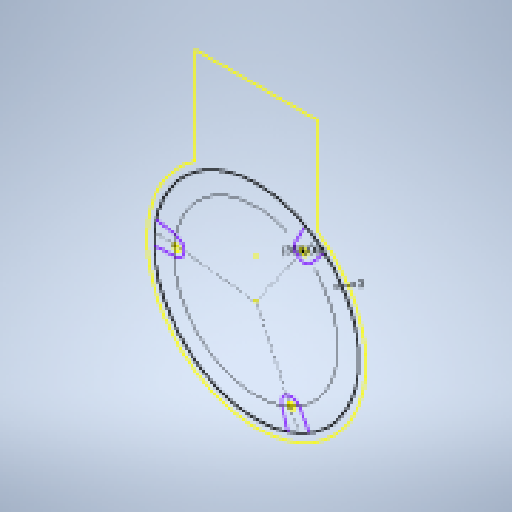
# Autodesk Inventor part: clips Anemo
Saved by Autodesk Inventor 2023 (Build 270158000, 158)
## iProperties
Created: 2023-03-28
Part Number: clips Anemo
Material: Générique
Document SubType Name: Modeling
Designer: eleves
Density: 1 g/cm^3
Appearance: Par défaut
Author: eleves
Autodesk Inventor part; units mm, degrees
ref_plane "YZ Plane" through (0, 0, 0) normal (1, 0, 0) x (0, 1, 0)
ref_plane "XZ Plane" through (0, 0, 0) normal (0, 1, 0) x (-1, 0, 0)
ref_plane "XY Plane" through (0, 0, 0) normal (0, 0, 1) x (1, 0, 0)
sketch "Esquisse1" plane through (0, 0, 0) normal (0, 0, 1) x (1, 0, 0)
  circle A0 centre (-32.9619, -13.3427) radius 1.5 projected
  circle A1 centre (14.3997, -46.0802) radius 1.5 projected
  circle A2 centre (19.4091, 11.459) radius 1.5 projected
  arc A3 (-25, 21.4166) -> (25, 21.4166) centre (0, -16) ccw projected
  line L0 (25, 61) -> (25, 21.4166) projected
  line L1 (-25, 61) -> (25, 61) projected
  line L2 (-25, 21.4166) -> (-25, 61) projected
  circle A4 centre (0, -16) radius 42
  line L3 (0, -16) -> (24.2426, 18.2972) construction
  arc A5 (15.8278, 13.0403) -> (22.2865, 8.8044) centre (19.4091, 11.459) ccw
  line L4 (22.2865, 8.8044) -> (28.0705, 15.2418)
  line L5 (15.8278, 13.0403) -> (20.0997, 20.8782)
  line L6 (0, -16) -> (-41.8235, -12.1539) construction
  arc A6 (-33.0635, -16.8129) -> (-32.6245, -9.1015) centre (-33.4847, -12.9207) ccw
  line L7 (-32.6245, -9.1015) -> (-41.0914, -7.3112)
  line L8 (-33.0635, -16.8129) -> (-41.9873, -17.0323)
  line L9 (0, -16) -> (17.5809, -54.1433) construction
  arc A7 (17.2357, -44.2274) -> (10.338, -47.7029) centre (14.0756, -46.5383) ccw
  line L10 (10.338, -47.7029) -> (13.021, -55.9306)
  line L11 (17.2357, -44.2274) -> (21.8876, -51.8459)
  circle A8 centre (0, -16) radius 45
  point P0 (0, 0)
  point P1 (25, 21.4166)
  point P2 (-25, 21.4166)
  dimension "d0" = 3
  dimension "d3" = 360
  constraints: 18 end point, 9 point on circle, 5 centre point, 5 coincident, 3 point on line, 2 line through centre, 37 other
  measures "d0" radial gap between concentric circles of A3 A4
extrude "Extrusion1" add sketch "Esquisse1" against normal blind 2 contours A8 A3 | L4 A5 L5 A4 | A4 L10 A7 L11 | L7 A6 L8 A4
sketch "Esquisse2" plane through (0, -16, -2) normal (0, 0, -1) x (-1, 0, 0)
  circle A0 centre (0, 0) radius 45
  point P0 (0, 16)
  constraints: 1 centre point
extrude "Extrusion2" add sketch "Esquisse2" along normal blind 2
